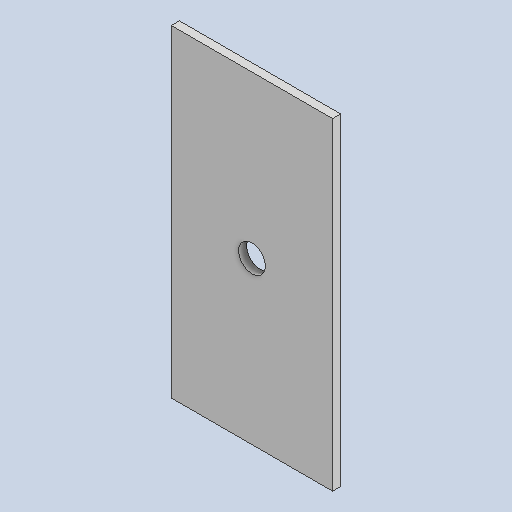
# Autodesk Inventor part: foot
Saved by Autodesk Inventor 2022 (Build 260153000, 153)
## iProperties
Created: 2022-10-09
Part Number: foot
Material: 一般
Document SubType Name: Modeling
Designer: haya
Density: 1 g/cm^3
Appearance: 既定
Author: haya
Autodesk Inventor part; units mm, degrees
ref_plane "YZ Plane" through (0, 0, 0) normal (1, 0, 0) x (0, 1, 0)
ref_plane "XZ Plane" through (0, 0, 0) normal (0, 1, 0) x (-1, 0, 0)
ref_plane "XY Plane" through (0, 0, 0) normal (0, 0, 1) x (1, 0, 0)
sketch "スケッチ1" plane through (0, 0, 0) normal (0, 0, 1) x (1, 0, 0)
  line L0 (0, 0) -> (60, 0)
  line L1 (60, 0) -> (60, 120)
  line L2 (60, 120) -> (0, 120)
  line L3 (0, 120) -> (0, 0)
  dimension "d0" = 60
  dimension "d1" = 120
  constraints: 8 end point, 2 parallel, 1 horizontal, 1 perpendicular
  measures "d0" distance of L0.start L0.end
  measures "d1" distance of L2.end L0.start
extrude "押し出し1" add sketch "スケッチ1" along normal blind 3
sketch "スケッチ2" plane through (0, 0, 3) normal (0, 0, 1) x (1, 0, 0)
  line L0 (60, 0) -> (60, 120) projected
  line L1 (60, 120) -> (0, 120) projected
  line L2 (0, 120) -> (0, 0) projected
  line L3 (0, 0) -> (60, 0) projected
  line L4 (30, 120) -> (30, 0) construction
  line L5 (0, 60) -> (60, 60) construction
  point P0 (30, 60)
  constraints: 5 midpoint, 4 end point
hole "穴1" at (30, 60, 3) direction (0, 0, -1) diameter 10 end through all
